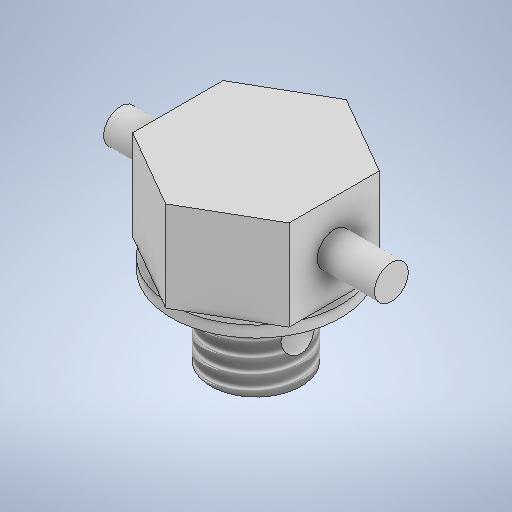
# Autodesk Inventor part: 123 cap
Saved by Autodesk Inventor 2025.1 (Build 291241000, 241)
## iProperties
Created: 2024-08-22
Part Number: 123 cap
Material: Generisch
Document SubType Name: Modeling
Designer: ffogue
Density: 1 g/cm^3
Appearance: Vorgabe
Author: ffogue
Autodesk Inventor part; units mm, degrees
sketch "Sketch1" plane through (0, 0, 0) normal (0, 0, 1) x (1, 0, 0)
  line L0 (0, 8) -> (6.9282, 4)
  line L1 (6.9282, 4) -> (6.9282, -4)
  line L2 (6.9282, -4) -> (0, -8)
  line L3 (0, -8) -> (-6.9282, -4)
  line L4 (-6.9282, -4) -> (-6.9282, 4)
  line L5 (-6.9282, 4) -> (0, 8)
  point P0 (0, 0)
  point P1 (0, 0)
  point P2 (-6.9282, 0)
  dimension "d0" = 16
  constraints: 12 end point, 1 coincident, 1 horizontal alignment, 1 midpoint, 13 other
  measures "d0" distance of L2.end L0.start
extrude "Extrusion1" add sketch "Sketch1" along normal blind 8
sketch "Sketch2" plane through (0, 0, 0) normal (0, 0, -1) x (-1, 0, 0)
  circle A0 centre (0, 0) radius 4
  dimension "d3" = 8
  constraints: 1 centre point, 1 coincident
  measures "d3" diameter of A0
extrude "Extrusion2" add sketch "Sketch2" along normal blind 8
sketch "Sketch3" plane through (0, 0, 0) normal (0, 0, -1) x (-1, 0, 0)
  circle A0 centre (0, 0) radius 7.5
  dimension "d6" = 15
  constraints: 1 centre point, 1 coincident
  measures "d6" diameter of A0
extrude "Extrusion3" add sketch "Sketch3" along normal blind 1
thread "Thread1" size "M8x1.25" class "6g" standard "ISO Metric profile" length 9.5
ref_plane "Work Plane1" through (7, 0, 0) normal (1, 0, 0) x (0, 1, 0)
sketch "Sketch4" plane through (7, 0, 0) normal (1, 0, 0) x (0, 1, 0)
  line L0 (-4, 8) -> (4, 8) projected
  line L1 (-2.8723, 0) -> (2.8723, 0) projected
  point P0 (0, 0)
  point P1 (0, 4)
  point P2 (0, 0)
  dimension "d12" = 4
  constraints: 1 midpoint, 1 vertical alignment
  measures "d12" distance from line of L0 point (0, 4)
hole "Hole1" at (7, 0, 4) direction (-1, 0, 0) diameter 3 end through all
ref_plane "Work Plane2" through (4, 0, 0) normal (1, 0, 0) x (0, 1, 0)
sketch "Sketch5" plane through (4, 0, 0) normal (1, 0, 0) x (0, 1, 0)
  line L0 (-2.8723, 0) -> (2.8723, 0) projected
  line L1 (-7.5, -1) -> (7.5, -1) projected
  point P0 (0, 0)
  point P1 (0, -4)
  point P2 (0, 0)
  dimension "d21" = 3
  constraints: 1 midpoint, 1 vertical alignment
  measures "d21" distance from line of L1 point (0, -4)
hole "Hole2" at (4, 0, -4) direction (-1, 0, 0) diameter 3 end through all
ref_plane "Work Plane3" through (0, 0, 0) normal (1, 0, 0) x (0, 1, 0)
sketch "Sketch6" plane through (0, 0, 0) normal (1, 0, 0) x (0, 1, 0)
  circle A0 centre (0, 4) radius 1.5 projected
  point P0 (0, 0)
extrude "Extrusion4" add sketch "Sketch6" along normal mid plane 24 separate body
body "Solid1"
